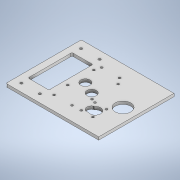
# Autodesk Inventor part: Port Support Plate
Saved by Autodesk Inventor 2021 (Build 250183000, 183)
## iProperties
Created: 2020-07-14
Part Number: Port Support Plate
Material: Generic
Document SubType Name: Modeling
Designer: jgray
Density: 1 g/cm^3
Appearance: Default
Author: jgray
Autodesk Inventor part; units mm, degrees
ref_plane "YZ Plane" through (0, 0, 0) normal (1, 0, 0) x (0, 1, 0)
ref_plane "XZ Plane" through (0, 0, 0) normal (0, 1, 0) x (-1, 0, 0)
ref_plane "XY Plane" through (0, 0, 0) normal (0, 0, 1) x (1, 0, 0)
sketch "Sketch1" plane through (0, 0, 0) normal (0, 1, 0) x (-1, 0, 0)
  line L0 (-16, -38) -> (16, -38)
  line L1 (18, -36) -> (18, 36)
  line L2 (16, 38) -> (-16, 38)
  line L3 (-18, 36) -> (-18, -36)
  line L4 (-18, -38) -> (18, 38) construction
  line L5 (18, -38) -> (-18, 38) construction
  line L6 (-16, -51.5) -> (16, -51.5) construction
  line L7 (16, -51.5) -> (16, 51.5) construction
  line L8 (16, 51.5) -> (-16, 51.5) construction
  line L9 (-16, 51.5) -> (-16, -51.5) construction
  line L10 (-16, -51.5) -> (16, 51.5) construction
  line L11 (16, -51.5) -> (-16, 51.5) construction
  line L12 (19.8993, 0) -> (-145.0451, 0) construction
  line L13 (-214, -65) -> (27, -65)
  line L14 (29, -63) -> (29, 63)
  line L15 (27, 65) -> (-214, 65)
  line L16 (-216, 63) -> (-216, -63)
  line L17 (-216, -65) -> (29, 65) construction
  line L18 (29, -65) -> (-216, 65) construction
  circle A0 centre (16, 51.5) radius 2.1
  circle A1 centre (16, -51.5) radius 2.1
  circle A2 centre (-16, -51.5) radius 2.1
  circle A3 centre (-16, 51.5) radius 2.1
  arc A4 (18, 36) -> (16, 38) centre (16, 36) ccw
  arc A5 (16, -38) -> (18, -36) centre (16, -36) ccw
  arc A6 (-18, -36) -> (-16, -38) centre (-16, -36) ccw
  arc A7 (-16, 38) -> (-18, 36) centre (-16, 36) ccw
  arc A8 (29, 63) -> (27, 65) centre (27, 63) ccw
  arc A9 (27, -65) -> (29, -63) centre (27, -63) ccw
  arc A10 (-216, -63) -> (-214, -65) centre (-214, -63) ccw
  arc A11 (-214, 65) -> (-216, 63) centre (-214, 63) ccw
  point P0 (0, 0)
  point P1 (-93.5, 0)
  dimension "d0" = 36
  dimension "d1" = 76
  dimension "d2" = 32
  dimension "d3" = 103
  dimension "d4" = 245
  dimension "d5" = 130
  dimension "d6" = 11
  dimension "d7" = 4.2
  dimension "d8" = 4.2
  dimension "d9" = 4.2
  dimension "d10" = 4.2
  dimension "d11" = 2
  dimension "d12" = 2
  constraints: 38 end point, 17 point on line, 16 point on circle, 16 tangent, 12 centre point, 8 coincident, 6 equal radius, 6 midpoint, 6 parallel, 4 horizontal, 3 perpendicular
  measures "d0" distance of L5.end L4.end
  measures "d1" distance of L4.end L5.start
  measures "d2" distance of L8.end L7.end
  measures "d3" distance of L7.end L6.end
  measures "d4" distance of L18.end L17.end
  measures "d5" distance of L17.end L18.start
  measures "d6" distance between parallel lines of L14 L1
  measures "d7" diameter of A0
  measures "d8" diameter of A1
  measures "d9" diameter of A2
  measures "d10" diameter of A3
  measures "d11" radius of A4
  measures "d12" radius of A8
extrude "Extrusion1" add sketch "Sketch1" along normal blind 5
sketch "Sketch2" plane through (0, 5, 0) normal (0, 1, 0) x (1, 0, 0)
  line L0 (-79.1767, 0) -> (130.5837, 0) construction
  line L1 (61, 41) -> (30, 41) construction
  line L2 (30, 41) -> (30, -41) construction
  line L3 (30, -41) -> (61, -41) construction
  line L4 (61, -41) -> (61, 41) construction
  line L5 (61, 41) -> (30, -41) construction
  line L6 (30, 41) -> (61, -41) construction
  line L7 (18, 36) -> (18, -36) construction
  point P0 (0, 0)
  point P1 (45.5, 0)
  dimension "d15" = 31
  dimension "d16" = 82
  dimension "d17" = 12
  constraints: 14 end point, 4 coincident, 2 horizontal, 2 midpoint, 2 parallel, 2 point on line, 1 perpendicular
  measures "d15" distance of L3.end L2.end
  measures "d16" distance of L2.end L1.end
  measures "d17" distance between parallel lines of L7 L2
hole "Hole1" at (30, 5, 41) at (30, 5, -41) at (61, 5, -41) at (61, 5, 41) direction (0, -1, 0) diameter 3.8 end through all
sketch "Sketch3" plane through (0, 5, 0) normal (0, 1, 0) x (1, 0, 0)
  line L0 (18, 36) -> (18, -36) projected
  line L1 (-62.6556, 0) -> (378.6556, 0) construction
  point P0 (0, 0)
  point P1 (18, 0)
  point P2 (108, 0)
  point P3 (158, 0)
  point P4 (193, 0)
  dimension "d0" = 36
  dimension "d1" = 76
  dimension "d4" = 245
  dimension "d5" = 130
  dimension "d6" = 11
  dimension "d11" = 2
  dimension "d12" = 2
  dimension "d25" = 90
  dimension "d26" = 140
  dimension "d27" = 175
  constraints: 3 point on line, 2 end point, 2 midpoint, 1 horizontal
  measures "d25" distance from line of L0 point (108, 0)
  measures "d26" distance from line of L0 point (158, 0)
  measures "d27" distance from line of L0 point (193, 0)
hole "Hole2" at (108, 5, 0) at (158, 5, 0) at (193, 5, 0) direction (0, -1, 0) diameter 27 end through all
sketch "Sketch4" plane through (0, 5, 0) normal (0, 1, 0) x (1, 0, 0)
  line L0 (67.1073, -17) -> (114.588, -17) construction
  line L1 (65.8182, -40.5) -> (127.5104, -40.5) construction
  line L2 (96.5, 60.0491) -> (96.5, 18.7989) construction
  line L3 (76.5, 60.0491) -> (76.5, 17.5099) construction
  line L4 (216, -63) -> (216, 63) projected
  line L5 (-27, -65) -> (214, -65) projected
  line L6 (214, 65) -> (-27, 65) projected
  point P0 (0, 0)
  point P1 (76.5, -17)
  point P2 (96.5, -17)
  point P3 (76.5, -40.5)
  point P4 (96.5, -40.5)
  dimension "d35" = 23.5
  dimension "d36" = 20
  dimension "d37" = 119.5
  dimension "d46" = 82
  constraints: 8 end point, 8 point on line, 2 horizontal, 2 vertical
  measures "d35" distance of point (96.5, -17) point (96.5, -40.5)
  measures "d36" distance between parallel lines of L2 L3
  measures "d37" distance between parallel lines of L4 L2
  measures "d46" distance between parallel lines of L6 L0
hole "Hole3" at (76.5, 5, 17) at (96.5, 5, 17) at (76.5, 5, 40.5) at (96.5, 5, 40.5) direction (0, -1, 0) diameter 3.8 end through all
sketch "Sketch5" plane through (0, 5, 0) normal (0, 1, 0) x (1, 0, 0)
  circle A0 centre (76.5, -40.5) radius 1.9 projected
  circle A1 centre (76.5, -17) radius 1.9 projected
  circle A2 centre (96.5, -17) radius 1.9 projected
  circle A3 centre (96.5, -40.5) radius 1.9 projected
  circle A4 centre (158, 0) radius 13.5 projected
  circle A5 centre (108, 0) radius 13.5 projected
  circle A6 centre (193, 0) radius 13.5 projected
  circle A7 centre (61, 41) radius 1.9 projected
  circle A8 centre (30, -41) radius 1.9 projected
  circle A9 centre (30, 41) radius 1.9 projected
  circle A10 centre (61, -41) radius 1.9 projected
  arc A11 (-27, 65) -> (-29, 63) centre (-27, 63) ccw projected
  line L0 (-29, 63) -> (-29, -63) projected
  arc A12 (-29, -63) -> (-27, -65) centre (-27, -63) ccw projected
  line L1 (-27, -65) -> (214, -65) projected
  arc A13 (214, -65) -> (216, -63) centre (214, -63) ccw projected
  line L2 (216, -63) -> (216, 63) projected
  arc A14 (216, 63) -> (214, 65) centre (214, 63) ccw projected
  line L3 (214, 65) -> (-27, 65) projected
  circle A15 centre (-16, -51.5) radius 2.1 projected
  circle A16 centre (-16, 51.5) radius 2.1 projected
  circle A17 centre (16, 51.5) radius 2.1 projected
  circle A18 centre (16, -51.5) radius 2.1 projected
  arc A19 (18, 36) -> (16, 38) centre (16, 36) ccw projected
  line L4 (18, 36) -> (18, -36) projected
  arc A20 (16, -38) -> (18, -36) centre (16, -36) ccw projected
  line L5 (16, -38) -> (-16, -38) projected
  arc A21 (-18, -36) -> (-16, -38) centre (-16, -36) ccw projected
  line L6 (-18, -36) -> (-18, 36) projected
  arc A22 (-16, 38) -> (-18, 36) centre (-16, 36) ccw projected
  line L7 (-16, 38) -> (16, 38) projected
  line L8 (81.2602, -23.5) -> (81.825, -23.5)
  line L9 (85.6801, -37.5) -> (81.2573, -37.5)
  arc A23 (81.2602, -23.5) -> (80.2232, -23.7899) centre (81.2602, -25.5) ccw
  arc A24 (80.1884, -37.1904) -> (81.2573, -37.5) centre (81.2573, -35.5) ccw
  arc A25 (85.6801, -37.5) -> (81.825, -23.5) centre (89.2, -29) ccw
  arc A26 (80.377, -23.7056) -> (80.4061, -37.3098) centre (84, -30.5) ccw
  point P0 (0, 0)
  point P1 (79.5, -23.5)
  point P2 (93.5, -23.5)
  dimension "d47" = 14
  dimension "d48" = 14
  dimension "d50" = 3
  dimension "d54" = 36
  dimension "d55" = 34.5
  dimension "d56" = 7.5
  dimension "d57" = 7.7
  dimension "d58" = 9.2
  dimension "d59" = 12.7
  constraints: 12 point on circle, 4 centre point, 4 end point, 2 point on line, 2 tangent, 1 equal radius, 1 horizontal, 1 parallel
  measures "d47" distance of point (79.5, -23.5) point (93.5, -23.5)
  measures "d48" distance between parallel lines of L8 L9
  measures "d50" distance from line of A3.centre L9
  measures "d54" distance from line of L1 A25.centre
  measures "d55" distance from line of L1 A26.centre
  measures "d56" horizontal distance of A0.centre A26.centre
  measures "d57" radius of A26
  measures "d58" radius of A25
  measures "d59" horizontal distance of A0.centre A25.centre
extrude "Extrusion2" cut sketch "Sketch5" against normal blind 10 contours L8 A25 L9 A24 A26 A23
sketch "Sketch6" plane through (0, 5, 0) normal (0, 1, 0) x (1, 0, 0)
  line L0 (27, 30.5) -> (69, 30.5) construction
  line L1 (69, 30.5) -> (69, -14.5) construction
  line L2 (69, -14.5) -> (27, -14.5) construction
  line L3 (27, -14.5) -> (27, 30.5) construction
  line L4 (-27, -65) -> (214, -65) construction
  line L5 (216, -63) -> (216, 63) construction
  line L6 (214, 65) -> (-27, 65) projected
  point P0 (0, 0)
  dimension "d60" = 42
  dimension "d61" = 45
  dimension "d63" = 147
  dimension "d71" = 34.5
  constraints: 8 end point, 4 coincident, 2 parallel, 1 horizontal, 1 perpendicular
  measures "d60" distance of L1.end L2.end
  measures "d61" distance of L0.end L1.end
  measures "d63" distance from line of L5 L1.end
  measures "d71" distance from line of L6 point (69, 30.5)
hole "Hole4" at (27, 5, -30.5) at (69, 5, -30.5) at (69, 5, 14.5) at (27, 5, 14.5) direction (0, -1, 0) diameter 3.8 end through all
sketch "Sketch7" plane through (0, 5, 0) normal (0, 1, 0) x (1, 0, 0)
  line L0 (-27, -65) -> (214, -65) projected
  line L1 (131, -65) -> (216, -65)
  line L2 (216, -65) -> (216, 65)
  line L3 (216, 65) -> (131, 65)
  line L4 (131, 65) -> (131, -65)
  line L5 (214, 65) -> (-27, 65) projected
  line L6 (216, -63) -> (216, 63) projected
  line L7 (-29, 63) -> (-29, -63) projected
  point P0 (0, 0)
  dimension "d72" = 160
  constraints: 8 end point, 2 collinear, 2 parallel, 1 horizontal, 1 perpendicular, 1 point on line
  measures "d72" distance between parallel lines of L4 L7
extrude "Extrusion3" cut sketch "Sketch7" against normal through all
sketch "Sketch9" plane through (0, 0, 0) normal (0, -1, 0) x (1, 0, 0)
  arc A0 (16, -38) -> (18, -36) centre (16, -36) ccw projected
  line L0 (-16, -38) -> (16, -38) projected
  arc A1 (-18, -36) -> (-16, -38) centre (-16, -36) ccw projected
  line L1 (-18, 36) -> (-18, -36) projected
  arc A2 (-16, 38) -> (-18, 36) centre (-16, 36) ccw projected
  line L2 (16, 38) -> (-16, 38) projected
  arc A3 (18, 36) -> (16, 38) centre (16, 36) ccw projected
  line L3 (18, -36) -> (18, 36) projected
  circle A4 centre (16, 51.5) radius 2.1 projected
  circle A5 centre (16, -51.5) radius 2.1 projected
  circle A6 centre (-16, -51.5) radius 2.1 projected
  circle A7 centre (-16, 51.5) radius 2.1 projected
  line L4 (131, -65) -> (131, 65) projected
  line L5 (-27, 65) -> (131, 65) projected
  arc A8 (-27, 65) -> (-29, 63) centre (-27, 63) ccw projected
  line L6 (-29, -63) -> (-29, 63) projected
  arc A9 (-29, -63) -> (-27, -65) centre (-27, -63) ccw projected
  line L7 (131, -65) -> (-27, -65) projected
  circle A10 centre (61, 41) radius 1.9 projected
  circle A11 centre (30, -41) radius 1.9 projected
  circle A12 centre (30, 41) radius 1.9 projected
  circle A13 centre (61, -41) radius 1.9 projected
  circle A14 centre (108, 0) radius 13.5 projected
  circle A15 centre (96.5, 40.5) radius 1.9 projected
  circle A16 centre (96.5, 17) radius 1.9 projected
  circle A17 centre (76.5, 17) radius 1.9 projected
  circle A18 centre (76.5, 40.5) radius 1.9 projected
  arc A19 (80.4061, 37.3098) -> (80.377, 23.7056) centre (84, 30.5) ccw projected
  arc A20 (81.2573, 37.5) -> (80.4061, 37.3098) centre (81.2573, 35.5) ccw projected
  line L8 (81.2573, 37.5) -> (85.6801, 37.5) projected
  arc A21 (81.825, 23.5) -> (85.6801, 37.5) centre (89.2, 29) ccw projected
  line L9 (81.825, 23.5) -> (81.2602, 23.5) projected
  arc A22 (80.377, 23.7056) -> (81.2602, 23.5) centre (81.2602, 25.5) ccw projected
  circle A23 centre (27, 14.5) radius 1.9 projected
  circle A24 centre (69, -30.5) radius 1.9 projected
  circle A25 centre (27, -30.5) radius 1.9 projected
  circle A26 centre (69, 14.5) radius 1.9 projected
  circle A27 centre (61, 7) radius 5.9 construction
  circle A28 centre (38.5, -4.5) radius 8
  line L10 (69, 14.5) -> (49.1378, -4.1208) construction
  circle A29 centre (59.468, 5.5637) radius 8
  line L11 (72.0115, 3.8809) -> (60.457, 16.2057) construction
  point P0 (0, 0)
  dimension "d75" = 7.5
  dimension "d76" = 8
  dimension "d77" = 11.5
  dimension "d78" = 19
  dimension "d79" = 11.8
  dimension "d80" = 16
  dimension "d81" = 16
  constraints: 4 end point, 3 centre point, 2 coincident, 2 point on line, 2 tangent, 1 perpendicular
  measures "d75" vertical distance of point (61, 7) L10.start
  measures "d76" horizontal distance of point (61, 7) L10.start
  measures "d77" horizontal distance of point (38.5, -4.5) A23.centre
  measures "d78" vertical distance of point (38.5, -4.5) A23.centre
  measures "d79" diameter of A27
  measures "d80" diameter of A28
  measures "d81" diameter of A29
extrude "Extrusion4" cut sketch "Sketch9" against normal through all contours A28 | A29
body "Solid1"
